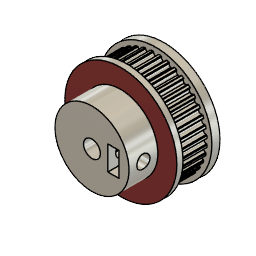
Polea_Motor_4mm_40T (Autodesk Fusion 360 design; units mm, degrees)
Autodesk Fusion 360 part; units mm, degrees
sketch "Sketch9" plane through (0, 0, 0) normal (0, 0, 1) x (1, 0, 0)
  circle A0 centre (0, 0) radius 12.4784
  circle A1 centre (0, 0) radius 11.7284
  line L0 (0, 0) -> (0, 12.4784) construction
  line L1 (0, 0) -> (12.4784, 0) construction
  circle A2 centre (0, 12.2834) radius 0.555
  line L2 (0, 0) -> (1.9521, 12.3248) construction
  circle A3 centre (1.9215, 12.1322) radius 0.555
  circle A4 centre (-0.7046, 12.3082) radius 0.15 construction
  circle A5 centre (0, 0) radius 2.5
  circle A6 centre (2.6213, 12.0465) radius 0.15 construction
  circle A7 centre (0.7046, 12.3082) radius 0.15
  circle A8 centre (1.2295, 12.2669) radius 0.15
  dimension "d124" = 24.9568
  dimension "d125" = -0.75
  dimension "d126" = 1.11
  dimension "d127" = 81
  dimension "d137" = 0.3
  dimension "d142" = 5
  dimension "d157" = 0.3
  constraint coincident A0.centre A1.centre
  constraint coincident A0 L0.end
  constraint vertical L0
  constraint coincident A0 L1.end
  constraint perpendicular L0 L1
  constraint coincident L0 A2.centre
  constraint tangent A1 A2
  constraint coincident A0 L2.end
  constraint coincident L2 A3.centre
  constraint equal A2 A3
  constraint tangent A1 A3
  constraint tangent A2 A4
  constraint tangent A0 A4
  constraint tangent A3 A6
  constraint tangent A0 A6
  constraint symmetric L0 A4 A7
  constraint symmetric L2 A6 A8
  measures "d124" diameter of A0
  measures "d126" diameter of A2
  measures "d127" angle of L1 L2
  measures "d137" diameter of A4
  measures "d142" diameter of A5
  measures "d157" diameter of A6
extrude "Extrude15" add sketch "Sketch9" along normal blind 7 contours A0 A1 A2 A3 A7 A8 | A8 | A7 makes body 1
pattern_circular "C-Pattern9" count 40 over 360 about axis through (0, 0, 1.75) along (0, 0, 1) of "Extrude15" makes body 2 at (-0.2047, 11.7266, 2.3333) makes body 3 at (-2.0366, 11.5502, 2.3333) makes body 4 at (-4.5826, 10.796, 4.6667) makes body 5 at (-6.2151, 9.9462, 4.6667) makes body 6 at (-7.6945, 8.8515, 4.6667) makes body 7 at (-8.4367, 8.1472, 2.3333) makes body 8 at (-9.6073, 6.7271, 2.3333) makes body 9 at (-10.5414, 5.1414, 2.3333) makes body 10 at (-11.2159, 3.4291, 2.3333) makes body 11 at (-11.6143, 1.6323, 2.3333) makes body 12 at (-11.7266, -0.2047, 2.3333) makes body 13 at (-11.5502, -2.0366, 2.3333) makes body 14 at (-10.796, -4.5826, 4.6667) makes body 15 at (-9.9462, -6.2151, 4.6667) makes body 16 at (-8.8515, -7.6945, 4.6667) makes body 17 at (-8.1472, -8.4367, 2.3333) makes body 18 at (-6.7271, -9.6073, 2.3333) makes body 19 at (-4.3935, -10.8744, 4.6667) makes body 20 at (-3.4291, -11.2159, 2.3333) makes body 21 at (-1.6323, -11.6143, 2.3333) makes body 22 at (0.2047, -11.7266, 2.3333) makes body 23 at (2.0366, -11.5502, 2.3333) makes body 24 at (3.8184, -11.0894, 2.3333) makes body 25 at (6.2151, -9.9462, 4.6667) makes body 26 at (7.6945, -8.8515, 4.6667) makes body 27 at (8.9845, -7.5389, 4.6667) makes body 28 at (9.6073, -6.7271, 2.3333) makes body 29 at (10.5414, -5.1414, 2.3333) makes body 30 at (11.2159, -3.4291, 2.3333) makes body 31 at (11.6143, -1.6323, 2.3333) makes body 32 at (11.7266, 0.2047, 2.3333) makes body 33 at (11.5502, 2.0366, 2.3333) makes body 34 at (11.0894, 3.8184, 2.3333) makes body 35 at (10.3556, 5.5061, 2.3333) makes body 36 at (8.8515, 7.6945, 4.6667) makes body 37 at (8.1472, 8.4367, 2.3333) makes body 38 at (6.0406, 10.0532, 4.6667) makes body 39 at (5.1414, 10.5414, 2.3333) makes body 40 at (3.4291, 11.2159, 2.3333)
extrude "Extrude16" add sketch "Sketch9" along normal up to surface (7 mm away) contours A1 bodies 1 2 3 4 5 6 7 8 9 10 11 12 13 14 15 16 17 18 19 20 21 22 23 24 25 26 27 28 29 30 31 32 33 34 35
sketch "Sketch10" plane through (0, 0, 7) normal (0, 0, 1) x (1, 0, 0)
  circle A0 centre (0, 0) radius 2.5
  arc A1 (1.2445, 12.4162) -> (0.7131, 12.458) centre (0, 0) ccw
  arc A2 (-0.5547, 12.303) -> (0.5547, 12.303) centre (0, 12.2834) ccw
  circle A3 centre (0, 0) radius 13.6015
  arc A4 (-0.7131, 12.458) -> (-1.2445, 12.4162) centre (0, 0) ccw
  arc A5 (-2.4724, 12.0647) -> (-1.3768, 12.2383) centre (-1.9215, 12.1322) ccw
  arc A6 (-2.6532, 12.1931) -> (-3.1715, 12.0686) centre (0, 0) ccw
  arc A7 (-4.3293, 11.5294) -> (-3.2743, 11.8722) centre (-3.7958, 11.6822) ccw
  arc A8 (-4.528, 11.6279) -> (-5.0204, 11.4239) centre (0, 0) ccw
  arc A9 (-6.0796, 10.7102) -> (-5.0912, 11.2138) centre (-5.5765, 10.9446) ccw
  arc A10 (-6.2912, 10.7764) -> (-6.7457, 10.4979) centre (0, 0) ccw
  arc A11 (-7.6802, 9.6273) -> (-6.7828, 10.2793) centre (-7.22, 9.9375) ccw
  arc A12 (-7.8996, 9.6596) -> (-8.3049, 9.3134) centre (0, 0) ccw
  arc A13 (-9.0917, 8.3073) -> (-8.3073, 9.0917) centre (-8.6857, 8.6857) ccw
  arc A14 (-9.3134, 8.3049) -> (-9.6596, 7.8996) centre (0, 0) ccw
  arc A15 (-10.2793, 6.7828) -> (-9.6273, 7.6802) centre (-9.9375, 7.22) ccw
  arc A16 (-10.4979, 6.7457) -> (-10.7764, 6.2912) centre (0, 0) ccw
  arc A17 (-11.2138, 5.0912) -> (-10.7102, 6.0796) centre (-10.9446, 5.5765) ccw
  arc A18 (-11.4239, 5.0204) -> (-11.6279, 4.528) centre (0, 0) ccw
  arc A19 (-11.8722, 3.2743) -> (-11.5294, 4.3293) centre (-11.6822, 3.7958) ccw
  arc A20 (-12.0686, 3.1715) -> (-12.1931, 2.6532) centre (0, 0) ccw
  arc A21 (-12.2383, 1.3768) -> (-12.0647, 2.4724) centre (-12.1322, 1.9215) ccw
  arc A22 (-12.4162, 1.2445) -> (-12.458, 0.7131) centre (0, 0) ccw
  arc A23 (-12.303, -0.5547) -> (-12.303, 0.5547) centre (-12.2834, 0) ccw
  arc A24 (-12.458, -0.7131) -> (-12.4162, -1.2445) centre (0, 0) ccw
  arc A25 (-12.0647, -2.4724) -> (-12.2383, -1.3768) centre (-12.1322, -1.9215) ccw
  arc A26 (-12.1931, -2.6532) -> (-12.0686, -3.1715) centre (0, 0) ccw
  arc A27 (-11.5294, -4.3293) -> (-11.8722, -3.2743) centre (-11.6822, -3.7958) ccw
  arc A28 (-11.6279, -4.528) -> (-11.4239, -5.0204) centre (0, 0) ccw
  arc A29 (-10.7102, -6.0796) -> (-11.2138, -5.0912) centre (-10.9446, -5.5765) ccw
  arc A30 (-10.7764, -6.2912) -> (-10.4979, -6.7457) centre (0, 0) ccw
  arc A31 (-9.6273, -7.6802) -> (-10.2793, -6.7828) centre (-9.9375, -7.22) ccw
  arc A32 (-9.6596, -7.8996) -> (-9.3134, -8.3049) centre (0, 0) ccw
  arc A33 (-8.3073, -9.0917) -> (-9.0917, -8.3073) centre (-8.6857, -8.6857) ccw
  arc A34 (-8.3049, -9.3134) -> (-7.8996, -9.6596) centre (0, 0) ccw
  arc A35 (-6.7828, -10.2793) -> (-7.6802, -9.6273) centre (-7.22, -9.9375) ccw
  arc A36 (-6.7457, -10.4979) -> (-6.2912, -10.7764) centre (0, 0) ccw
  arc A37 (-5.0912, -11.2138) -> (-6.0796, -10.7102) centre (-5.5765, -10.9446) ccw
  arc A38 (-5.0204, -11.4239) -> (-4.528, -11.6279) centre (0, 0) ccw
  arc A39 (-3.2743, -11.8722) -> (-4.3293, -11.5294) centre (-3.7958, -11.6822) ccw
  arc A40 (-3.1715, -12.0686) -> (-2.6532, -12.1931) centre (0, 0) ccw
  arc A41 (-1.3768, -12.2383) -> (-2.4724, -12.0647) centre (-1.9215, -12.1322) ccw
  arc A42 (-1.2445, -12.4162) -> (-0.7131, -12.458) centre (0, 0) ccw
  arc A43 (0.5547, -12.303) -> (-0.5547, -12.303) centre (0, -12.2834) ccw
  arc A44 (0.7131, -12.458) -> (1.2445, -12.4162) centre (0, 0) ccw
  arc A45 (2.4724, -12.0647) -> (1.3768, -12.2383) centre (1.9215, -12.1322) ccw
  arc A46 (2.6532, -12.1931) -> (3.1715, -12.0686) centre (0, 0) ccw
  arc A47 (4.3293, -11.5294) -> (3.2743, -11.8722) centre (3.7958, -11.6822) ccw
  arc A48 (4.528, -11.6279) -> (5.0204, -11.4239) centre (0, 0) ccw
  arc A49 (6.0796, -10.7102) -> (5.0912, -11.2138) centre (5.5765, -10.9446) ccw
  arc A50 (6.2912, -10.7764) -> (6.7457, -10.4979) centre (0, 0) ccw
  arc A51 (7.6802, -9.6273) -> (6.7828, -10.2793) centre (7.22, -9.9375) ccw
  arc A52 (7.8996, -9.6596) -> (8.3049, -9.3134) centre (0, 0) ccw
  arc A53 (9.0917, -8.3073) -> (8.3073, -9.0917) centre (8.6857, -8.6857) ccw
  arc A54 (9.3134, -8.3049) -> (9.6596, -7.8996) centre (0, 0) ccw
  arc A55 (10.2793, -6.7828) -> (9.6273, -7.6802) centre (9.9375, -7.22) ccw
  arc A56 (10.4979, -6.7457) -> (10.7764, -6.2912) centre (0, 0) ccw
  arc A57 (11.2138, -5.0912) -> (10.7102, -6.0796) centre (10.9446, -5.5765) ccw
  arc A58 (11.4239, -5.0204) -> (11.6279, -4.528) centre (0, 0) ccw
  arc A59 (11.8722, -3.2743) -> (11.5294, -4.3293) centre (11.6822, -3.7958) ccw
  arc A60 (12.0686, -3.1715) -> (12.1931, -2.6532) centre (0, 0) ccw
  arc A61 (12.2383, -1.3768) -> (12.0647, -2.4724) centre (12.1322, -1.9215) ccw
  arc A62 (12.4162, -1.2445) -> (12.458, -0.7131) centre (0, 0) ccw
  arc A63 (12.303, 0.5547) -> (12.303, -0.5547) centre (12.2834, 0) ccw
  arc A64 (12.458, 0.7131) -> (12.4162, 1.2445) centre (0, 0) ccw
  arc A65 (12.0647, 2.4724) -> (12.2383, 1.3768) centre (12.1322, 1.9215) ccw
  arc A66 (12.1931, 2.6532) -> (12.0686, 3.1715) centre (0, 0) ccw
  arc A67 (11.5294, 4.3293) -> (11.8722, 3.2743) centre (11.6822, 3.7958) ccw
  arc A68 (11.6279, 4.528) -> (11.4239, 5.0204) centre (0, 0) ccw
  arc A69 (10.7102, 6.0796) -> (11.2138, 5.0912) centre (10.9446, 5.5765) ccw
  arc A70 (10.7764, 6.2912) -> (10.4979, 6.7457) centre (0, 0) ccw
  arc A71 (9.4885, 6.8938) -> (10.2793, 6.7828) centre (9.9375, 7.22) ccw
  arc A72 (-6.7828, -10.2793) -> (-6.7457, -10.4979) centre (-6.6646, -10.3717) ccw
  arc A73 (-6.2912, -10.7764) -> (-6.0796, -10.7102) centre (-6.2156, -10.6469) ccw
  arc A74 (-5.0912, -11.2138) -> (-5.0204, -11.4239) centre (-4.9601, -11.2866) ccw
  arc A75 (-4.528, -11.6279) -> (-4.3293, -11.5294) centre (-4.4735, -11.4881) ccw
  arc A76 (-3.2743, -11.8722) -> (-3.1715, -12.0686) centre (-3.1334, -11.9236) ccw
  arc A77 (-2.6532, -12.1931) -> (-2.4724, -12.0647) centre (-2.6213, -12.0465) ccw
  arc A78 (-1.3768, -12.2383) -> (-1.2445, -12.4162) centre (-1.2295, -12.2669) ccw
  arc A79 (-0.7131, -12.458) -> (-0.5547, -12.303) centre (-0.7046, -12.3082) ccw
  arc A80 (0.5547, -12.303) -> (0.7131, -12.458) centre (0.7046, -12.3082) ccw
  arc A81 (1.2445, -12.4162) -> (1.3768, -12.2383) centre (1.2295, -12.2669) ccw
  arc A82 (2.4724, -12.0647) -> (2.6532, -12.1931) centre (2.6213, -12.0465) ccw
  arc A83 (3.1715, -12.0686) -> (3.2743, -11.8722) centre (3.1334, -11.9236) ccw
  arc A84 (4.3293, -11.5294) -> (4.528, -11.6279) centre (4.4735, -11.4881) ccw
  arc A85 (5.0204, -11.4239) -> (5.0912, -11.2138) centre (4.9601, -11.2866) ccw
  arc A86 (6.0796, -10.7102) -> (6.2912, -10.7764) centre (6.2156, -10.6469) ccw
  arc A87 (6.7457, -10.4979) -> (6.7828, -10.2793) centre (6.6646, -10.3717) ccw
  arc A88 (7.6802, -9.6273) -> (7.8996, -9.6596) centre (7.8046, -9.5434) ccw
  arc A89 (8.3049, -9.3134) -> (8.3073, -9.0917) centre (8.205, -9.2014) ccw
  arc A90 (9.0917, -8.3073) -> (9.3134, -8.3049) centre (9.2014, -8.205) ccw
  arc A91 (9.6596, -7.8996) -> (9.6273, -7.6802) centre (9.5434, -7.8046) ccw
  arc A92 (10.2793, -6.7828) -> (10.4979, -6.7457) centre (10.3717, -6.6646) ccw
  arc A93 (10.7764, -6.2912) -> (10.7102, -6.0796) centre (10.6469, -6.2156) ccw
  arc A94 (11.2138, -5.0912) -> (11.4239, -5.0204) centre (11.2866, -4.9601) ccw
  arc A95 (11.6279, -4.528) -> (11.5294, -4.3293) centre (11.4881, -4.4735) ccw
  arc A96 (11.8722, -3.2743) -> (12.0686, -3.1715) centre (11.9236, -3.1334) ccw
  arc A97 (12.1931, -2.6532) -> (12.0647, -2.4724) centre (12.0465, -2.6213) ccw
  arc A98 (12.2383, -1.3768) -> (12.4162, -1.2445) centre (12.2669, -1.2295) ccw
  arc A99 (12.458, -0.7131) -> (12.303, -0.5547) centre (12.3082, -0.7046) ccw
  arc A100 (12.303, 0.5547) -> (12.458, 0.7131) centre (12.3082, 0.7046) ccw
  arc A101 (12.4162, 1.2445) -> (12.2383, 1.3768) centre (12.2669, 1.2295) ccw
  arc A102 (12.0647, 2.4724) -> (12.1931, 2.6532) centre (12.0465, 2.6213) ccw
  arc A103 (12.0686, 3.1715) -> (11.8722, 3.2743) centre (11.9236, 3.1334) ccw
  arc A104 (11.5294, 4.3293) -> (11.6279, 4.528) centre (11.4881, 4.4735) ccw
  arc A105 (11.4239, 5.0204) -> (11.2138, 5.0912) centre (11.2866, 4.9601) ccw
  arc A106 (10.7102, 6.0796) -> (10.7764, 6.2912) centre (10.6469, 6.2156) ccw
  arc A107 (10.4979, 6.7457) -> (10.2793, 6.7828) centre (10.3717, 6.6646) ccw
  arc A108 (1.3768, 12.2383) -> (1.2445, 12.4162) centre (1.2295, 12.2669) ccw
  arc A109 (0.7131, 12.458) -> (0.5547, 12.303) centre (0.7046, 12.3082) ccw
  arc A110 (-0.5547, 12.303) -> (-0.7131, 12.458) centre (-0.7046, 12.3082) ccw
  arc A111 (-1.2445, 12.4162) -> (-1.3768, 12.2383) centre (-1.2295, 12.2669) ccw
  arc A112 (-2.4724, 12.0647) -> (-2.6532, 12.1931) centre (-2.6213, 12.0465) ccw
  arc A113 (-3.1715, 12.0686) -> (-3.2743, 11.8722) centre (-3.1334, 11.9236) ccw
  arc A114 (-4.3293, 11.5294) -> (-4.528, 11.6279) centre (-4.4735, 11.4881) ccw
  arc A115 (-5.0204, 11.4239) -> (-5.0912, 11.2138) centre (-4.9601, 11.2866) ccw
  arc A116 (-6.0796, 10.7102) -> (-6.2912, 10.7764) centre (-6.2156, 10.6469) ccw
  arc A117 (-6.7457, 10.4979) -> (-6.7828, 10.2793) centre (-6.6646, 10.3717) ccw
  arc A118 (-7.6802, 9.6273) -> (-7.8996, 9.6596) centre (-7.8046, 9.5434) ccw
  arc A119 (-8.3049, 9.3134) -> (-8.3073, 9.0917) centre (-8.205, 9.2014) ccw
  arc A120 (-9.0917, 8.3073) -> (-9.3134, 8.3049) centre (-9.2014, 8.205) ccw
  arc A121 (-9.6596, 7.8996) -> (-9.6273, 7.6802) centre (-9.5434, 7.8046) ccw
  arc A122 (-10.2793, 6.7828) -> (-10.4979, 6.7457) centre (-10.3717, 6.6646) ccw
  arc A123 (-10.7764, 6.2912) -> (-10.7102, 6.0796) centre (-10.6469, 6.2156) ccw
  arc A124 (-11.2138, 5.0912) -> (-11.4239, 5.0204) centre (-11.2866, 4.9601) ccw
  arc A125 (-11.6279, 4.528) -> (-11.5294, 4.3293) centre (-11.4881, 4.4735) ccw
  arc A126 (-11.8722, 3.2743) -> (-12.0686, 3.1715) centre (-11.9236, 3.1334) ccw
  arc A127 (-12.1931, 2.6532) -> (-12.0647, 2.4724) centre (-12.0465, 2.6213) ccw
  arc A128 (-12.2383, 1.3768) -> (-12.4162, 1.2445) centre (-12.2669, 1.2295) ccw
  arc A129 (-12.458, 0.7131) -> (-12.303, 0.5547) centre (-12.3082, 0.7046) ccw
  arc A130 (-12.303, -0.5547) -> (-12.458, -0.7131) centre (-12.3082, -0.7046) ccw
  arc A131 (-12.4162, -1.2445) -> (-12.2383, -1.3768) centre (-12.2669, -1.2295) ccw
  arc A132 (-12.0647, -2.4724) -> (-12.1931, -2.6532) centre (-12.0465, -2.6213) ccw
  arc A133 (-12.0686, -3.1715) -> (-11.8722, -3.2743) centre (-11.9236, -3.1334) ccw
  arc A134 (-11.5294, -4.3293) -> (-11.6279, -4.528) centre (-11.4881, -4.4735) ccw
  arc A135 (-11.4239, -5.0204) -> (-11.2138, -5.0912) centre (-11.2866, -4.9601) ccw
  arc A136 (-10.7102, -6.0796) -> (-10.7764, -6.2912) centre (-10.6469, -6.2156) ccw
  arc A137 (-10.4979, -6.7457) -> (-10.2793, -6.7828) centre (-10.3717, -6.6646) ccw
  arc A138 (-9.6273, -7.6802) -> (-9.6596, -7.8996) centre (-9.5434, -7.8046) ccw
  arc A139 (-9.3134, -8.3049) -> (-9.0917, -8.3073) centre (-9.2014, -8.205) ccw
  arc A140 (-8.3073, -9.0917) -> (-8.3049, -9.3134) centre (-8.205, -9.2014) ccw
  arc A141 (-7.8996, -9.6596) -> (-7.6802, -9.6273) centre (-7.8046, -9.5434) ccw
  arc A142 (9.4885, 6.8938) -> (1.8347, 11.584) centre (0, 0) ccw
  arc A143 (1.3768, 12.2383) -> (1.8347, 11.584) centre (1.9215, 12.1322) ccw
  dimension "d156" = 27.2029
  constraint coincident A0.centre A1.centre
  measures "d156" diameter of A3
extrude "Extrude17" add sketch "Sketch10" along normal blind 1.5 contours A1 A2 A4 A5 A6 A7 A8 A9 A10 A11 A12 A13 A14 A15 A16 A17 A18 A19 A20 A21 A22 A23 A24 A25 A26 A27 A28 A29 A30 A31 A32 A33 A34 A35 A36 A37 A38 A39 A40 A41 A42 A43 A44 A45 A46 A47 A48 A49 A50 A51 A52 A53 A54 A55 A56 A57 A58 A59 A60 A61 A62 A63 A64 A65 A66 A67 A68 A69 A70 A71 A72 A73 A74 A75 A76 A77 A78 A79 A80 A81 A82 A83 A84 A85 A86 A87 A88 A89 A90 A91 A92 A93 A94 A95 A96 A97 A98 A99 A100 A101 A102 A103 A104 A105 A106 A107 A108 A109 A110 A111 A112 A113 A114 A115 A116 A117 A118 A119 A120 A121 A122 A123 A124 A125 A126 A127 A128 A129 A130 A131 A132 A133 A134 A135 A136 A137 A138 A139 A140 A141 A142 A143 | A3 bodies 1
extrude "Extrude18" add sketch "Sketch10" against normal blind 2 from surface at -7 contours A1 A2 A4 A5 A6 A7 A8 A9 A10 A11 A12 A13 A14 A15 A16 A17 A18 A19 A20 A21 A22 A23 A24 A25 A26 A27 A28 A29 A30 A31 A32 A33 A34 A35 A36 A37 A38 A39 A40 A41 A42 A43 A44 A45 A46 A47 A48 A49 A50 A51 A52 A53 A54 A55 A56 A57 A58 A59 A60 A61 A62 A63 A64 A65 A66 A67 A68 A69 A70 A71 A72 A73 A74 A75 A76 A77 A78 A79 A80 A81 A82 A83 A84 A85 A86 A87 A88 A89 A90 A91 A92 A93 A94 A95 A96 A97 A98 A99 A100 A101 A102 A103 A104 A105 A106 A107 A108 A109 A110 A111 A112 A113 A114 A115 A116 A117 A118 A119 A120 A121 A122 A123 A124 A125 A126 A127 A128 A129 A130 A131 A132 A133 A134 A135 A136 A137 A138 A139 A140 A141 A142 A143 | A3 bodies 1
sketch "Sketch12" plane through (0, 0, -2) normal (0, 0, -1) x (-1, 0, 0)
  circle A0 centre (0, 0) radius 2.5
  circle A1 centre (0, 0) radius 13.6015
  circle A2 centre (0, 0) radius 28.2
  dimension "d158" = 56.4
  constraint coincident A0.centre A1.centre
  measures "d158" diameter of A2
sketch "Sketch13" plane through (0, 0, 8.5) normal (0, 0, 1) x (1, 0, 0)
  circle A0 centre (0, 0) radius 2.5
  circle A1 centre (0, 0) radius 13.6015
  circle A2 centre (0, 0) radius 9
  circle A3 centre (0, 0) radius 2.05
  circle A4 centre (0, 0) radius 11
  dimension "d165" = 18
  dimension "d166" = 4.1
  constraint coincident A0.centre A1.centre
  constraint concentric A2 A3
  measures "d165" diameter of A2
  measures "d166" diameter of A3
extrude "Extrude23" add sketch "Sketch13" along normal blind 7 contours A0 | A2 bodies 1
sketch "Sketch14" plane through (0, 0, 15.5) normal (0, 0, 1) x (1, 0, 0)
  circle A0 centre (0, 0) radius 2.05
  circle A1 centre (0, 0) radius 2.55
  line L0 (0, 0) -> (5.2, 0)
  line L1 (6.55, -2.95) -> (3.85, -2.95)
  line L2 (3.85, -2.95) -> (3.85, 2.95)
  line L3 (3.85, 2.95) -> (6.55, 2.95)
  line L4 (6.55, 2.95) -> (6.55, -2.95)
  line L5 (6.55, -2.95) -> (3.85, 2.95) construction
  line L6 (3.85, -2.95) -> (6.55, 2.95) construction
  circle A2 centre (0, 0) radius 9
  point P0 (5.2, 0)
  dimension "d172" = 2.7
  dimension "d173" = 5.9
  constraint coincident A0.centre A1.centre
  constraint horizontal L0
  constraint horizontal L1
  constraint perpendicular L1 L2
  constraint parallel L1 L3
  constraint parallel L2 L4
  constraint coincident L5 P0
  constraint coincident L6 P0
  constraint coincident P0 L0.end
  measures "d172" distance of L2.end L3.end
  measures "d173" distance of L1.end L2.end
extrude "Extrude25" cut sketch "Sketch14" against normal blind 5.117 contours L1 L2 L3 L4 bodies 1
sketch "Sketch15" plane through (3.85, 0, 0) normal (1, 0, 0) x (0, 0, -1)
  line L0 (-15.5, 2.95) -> (-15.5, -2.95)
  line L1 (-15.5, -2.95) -> (-10.383, -2.95)
  line L2 (-10.383, -2.95) -> (-10.383, 2.95)
  line L3 (-10.383, 2.95) -> (-15.5, 2.95)
  line L4 (-15.5, 0) -> (-12, 0)
  line L5 (-10.3834, -2.8) -> (-8.7668, 0)
  line L6 (-8.7668, 0) -> (-10.3834, 2.8)
  line L7 (-10.3834, 2.8) -> (-13.6166, 2.8)
  line L8 (-13.6166, 2.8) -> (-15.2332, 0)
  line L9 (-15.2332, 0) -> (-13.6166, -2.8)
  line L10 (-13.6166, -2.8) -> (-10.3834, -2.8)
  circle A0 centre (-12, 0) radius 1.6
  line L11 (-10.3834, 2.8) -> (-10.3834, -2.8)
  point P0 (-12, 0)
  dimension "d176" = 3.5
  dimension "d177" = 2.8
  dimension "d178" = 3.2
  constraint midpoint L0 L4.start
  constraint perpendicular L2 L4
  constraint coincident P0 L4.end
  measures "d176" distance of L4.start P0
  measures "d177" distance of P0 L10
  measures "d178" diameter of A0
extrude "Extrude26" cut sketch "Sketch15" against normal blind 3 contours A0 bodies 1
extrude "Extrude27" cut sketch "Sketch15" along normal blind 29 contours A0 bodies 1
extrude "Extrude28" cut sketch "Sketch15" along normal blind 2.6 contours L2 L5 L6 L11 bodies 1
extrude "Extruir29" add sketch "Sketch14" against normal up to surface (17.5 mm away) contours A1 bodies 1
sketch "Boceto18" plane through (0, 0, 15.5) normal (0, 0, 1) x (1, 0, 0)
  circle A0 centre (0, 0) radius 2.05
  line L0 (3.85, -2.95) -> (3.85, 2.95)
  line L1 (3.85, 2.95) -> (6.55, 2.95)
  line L2 (6.55, 2.95) -> (6.55, -2.95)
  line L3 (6.55, -2.95) -> (3.85, -2.95)
  circle A1 centre (0, 0) radius 9
  circle A2 centre (0, 0) radius 11
  constraint coincident A0.centre A1.centre
equation "OD_ = PD_ - ( 2 * U_ )" comment "Outer diameter"
equation "PD_ = ( ( P_ * N_ ) / PI )" comment "Pitch Diameter"
equation "U_ = 0.254 mm" comment "Distance between the tensile cord and the bottom of the timming belt tooth, also called PLD"
equation "H_ = -0.75 mm" comment "distance between pulley tooth and belt tooth"
equation "P_ = 2 mm" comment "Pitch of the system"
equation "BTD_ = 0.555 mm * 2" comment "Belt tooth diameter"
equation "N_ = 40" comment "Number of teeth in the circumference pulley"
equation "PTR_ = ( 0.15 * 2 ) * 1 mm" comment "Pulley tooth roundness"
equation "EX_ = 7 mm" comment "Tooth Extrude length"
equation "SHFT_ = 5 mm" comment "The shaft diameter"
equation "TH_ = 90 deg - ( ( 360 / N_ ) * 1 deg )" comment "Radial distance between teeth"
equation "d124 = OD_"
equation "d125 = H_"
equation "d126 = BTD_"
equation "d127 = TH_"
equation "d137 = PTR_"
equation "d138 = EX_"
equation "d140 = N_"
equation "d142 = SHFT_"
equation "d156 = OD_ * 1.09"
